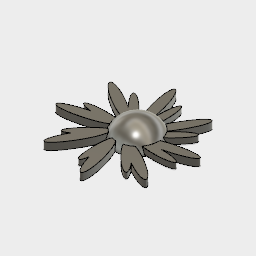
花瓣 v5 (Autodesk Fusion 360 design; units mm, degrees)
Autodesk Fusion 360 part; units mm, degrees
sketch "草图1" plane through (0, 0, 0) normal (0, 1, 0) x (1, 0, 0)
  ellipse E0 centre (0, 0) end of major axis (10, 0) minor radius 2
  line L0 (-10, 0) -> (10, 0)
  line L1 (0, -2) -> (0, 2)
extrude "拉伸1" add sketch "草图1" along normal blind 3 makes body 1
move_body "移动1" bodies 1 to x (0.965926, 0, -0.258819) y (0, 1, 0) z (0.258819, 0, 0.965926) at (0.1769, 0, -2.6563)
box "长方体基本要素1" add length 5 width 5 height 5 placed x (0, 0, -1) y (-1, 0, 0) z (0, 1, 0) at (-15, 0, 0) separate body makes body 2
pattern_circular "C-阵列1" count 8 over 360 about axis through (-15, 5, 0) along (0, -1, 0) of bodies 1 makes body 3 at (-0.5308, 0, 10.6174) makes body 4 at (-12.2764, 0, 17.7389) makes body 5 at (-25.6174, 0, 14.4692) makes body 6 at (-32.7389, 0, 2.7236) makes body 7 at (-29.4692, 0, -10.6174) makes body 8 at (-17.5891, 0, -12.6149) makes body 9 at (-7.9107, 0, -10.7508)
copy_body "复制和粘贴实体1" bodies 1 3 4 5 6 7 8 9 makes body 10 makes body 11 makes body 12 makes body 13 makes body 14 makes body 15 makes body 16 makes body 17
scale "缩放1" factor 0.8 about (-9.4824, 3, -0.0681) bodies 10 11 12 13 14 15 16 17
move_body "移动2" bodies 10 11 12 13 14 15 16 17 2 to x (0.965926, 0, 0.258819) y (0, 1, 0) z (-0.258819, 0, 0.965926) at (-0.5111, 0, 3.8823)
sphere "球体基本要素1" add diameter 20 placed x (1, 0, 0) y (0, 0, -1) z (0, 1, 0) at (-13.5, 0, -2.5) separate body makes body 18
move_body "MoveFace1" bodies 18 to x (1, 0, 0) y (0, 1, 0) z (0, 0, 1) at (0, -2, 0) on bodies 18
combine "合并1" operation add target body 18 tool bodies 1 3 4 5 6 7 8 9 10 11 17 16 15 14 13 12
box "长方体基本要素2" cut length 74 width 66 height -12 placed x (0, 0, -1) y (-1, 0, 0) z (0, 1, 0) at (29, 0, 47) bodies 18
hidden bodies 2
